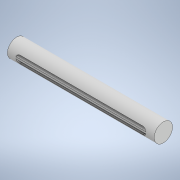
# Autodesk Inventor part: Inner_telescope_arm
Saved by Autodesk Inventor 2020 (Build 240168000, 168)
## iProperties
Created: 2019-08-27
Part Number: Inner_telescope_arm
Material: 常规
Document SubType Name: Modeling
Designer: User
Density: 1 g/cm^3
Appearance: 默认
Author: User
Autodesk Inventor part; units mm, degrees
ref_plane "XZ Plane" through (0, 0, 0) normal (0, 1, 0) x (-1, 0, 0)
ref_plane "XY Plane" through (0, 0, 0) normal (0, 0, 1) x (1, 0, 0)
sketch "草图1" plane through (0, 0, 0) normal (1, 0, 0) x (0, 1, 0)
  circle A0 centre (0, 0) radius 5
  dimension "d0" = 10
  constraints: 1 centre point, 1 coincident
  measures "d0" diameter of A0
extrude "拉伸1" add sketch "草图1" along normal blind 80
ref_plane "工作平面1" through (2.5, 0, 0) normal (1, 0, 0) x (0, 1, 0)
sketch "草图2" plane through (2.5, 0, 0) normal (1, 0, 0) x (0, 1, 0)
  circle A0 centre (0, 0) radius 5 projected
  line L0 (4, -1.7128) -> (-4, -1.7128)
  line L1 (-4, -1.7128) -> (-4, 1.7872)
  line L2 (-4, 1.7872) -> (4, 1.7872)
  line L3 (4, 1.7872) -> (4, -1.7128)
  line L4 (6.59, 0.0372) -> (-6.5609, 0.0372)
  point P0 (5, 0)
  point P1 (-5, 0)
  dimension "d4" = 1
  dimension "d5" = 1
  dimension "d6" = 3.5
  constraints: 10 end point, 2 horizontal, 2 parallel, 2 point on circle, 1 perpendicular, 1 other
  measures "d4" distance from line of A0.start L3
  measures "d5" distance from line of A0.end L1
  measures "d6" distance of L2.end L0.start
extrude "拉伸2" cut sketch "草图2" along normal blind 75 contours L4 L1 L2 L3 | L3 L0 L1 L4
ref_plane "工作平面3" through (0, 0, 5) normal (0, 0, 1) x (1, 0, 0)
sketch "草图5" plane through (0, 0, 5) normal (0, 0, 1) x (1, 0, 0)
  line L0 (-2.1953, 0) -> (98.9957, 0)
  line L1 (2.5, 4) -> (2.5, -4) projected
  line L2 (77.5, 4) -> (77.5, -4) projected
  line L3 (6.5, -2) -> (73.5, -2)
  line L4 (73.5, 2) -> (6.5, 2)
  arc A0 (73.5, -2) -> (73.5, 2) centre (73.5, 0) ccw
  arc A1 (6.5, 2) -> (6.5, -2) centre (6.5, 0) ccw
  line L5 (4.5635, 0.5) -> (75.4365, 0.5)
  line L6 (75.4365, -0.5) -> (4.5635, -0.5)
  point P0 (0, 0)
  point P1 (4.5, -2)
  point P2 (4.5, 2)
  point P3 (75, 0)
  point P4 (75.5, 0)
  point P5 (5, 0)
  point P6 (4.5, 0)
  dimension "d9" = 4
  dimension "d12" = 2
  dimension "d15" = 0.5
  dimension "d16" = 0.5
  constraints: 11 point on circle, 10 end point, 5 point on line, 4 horizontal, 2 centre point, 2 coincident, 2 parallel, 1 other
  measures "d9" distance between parallel lines of L4 L3
  measures "d12" distance from line of point (75.5, 0) L2
  measures "d15" distance of point (75.5, 0) point (75, 0)
  measures "d16" distance of point (5, 0) point (4.5, 0)
extrude "拉伸3" cut sketch "草图5" against normal blind 4 contours A1 L4 A0 L5 | L6 A0 L3 A1
